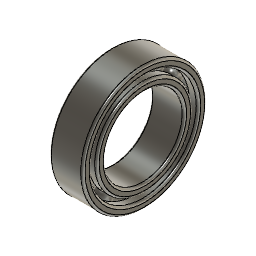
final (Autodesk Fusion 360 archive; units mm, degrees)
design "mr117zz"
Autodesk Fusion 360 part; units mm, degrees
sketch "Sketch1" plane through (0, 0, 0) normal (0, 0, 1) x (1, 0, 0)
  line L0 (-1.5, 3.5) -> (1.5, 3.5)
  line L1 (1.5, 3.5) -> (1.5, 4.25)
  line L2 (1.5, 4.25) -> (-1.5, 4.25)
  line L3 (-1.5, 4.25) -> (-1.5, 3.5)
  line L4 (-1.5, 5.5) -> (1.5, 5.5)
  line L5 (1.5, 5.5) -> (1.5, 4.75)
  line L6 (1.5, 4.75) -> (-1.5, 4.75)
  line L7 (-1.5, 4.75) -> (-1.5, 5.5)
  circle A0 centre (0, 4.5) radius 0.75
  line L8 (0, 3.5) -> (0, 5.5)
  line L9 (0, 3.5) -> (0, 0) construction
  dimension "d1" = 3
  dimension "d2" = 3.5
  dimension "d3" = 5.5
  dimension "d4" = 1.5
  dimension "d5" = 0.75
  constraint horizontal L0
  constraint vertical L1
  constraint horizontal L2
  constraint vertical L3
  constraint horizontal L4
  constraint vertical L5
  constraint horizontal L6
  constraint vertical L7
  constraint equal L0 L4
  constraint midpoint L0 L8.start
  constraint midpoint L4 L8.end
  constraint vertical L8
  constraint midpoint A0.centre L8
  constraint coincident L9.end origin
  constraint collinear L8 L9
  constraint equal L3 L7
  measures "d1" distance of L0.start L0.end
  measures "d2" distance of L9.end L0
  measures "d3" distance of L9.end L4
  measures "d4" diameter of A0
  measures "d5" distance of L0.start L2.end
revolve "Revolve1" add sketch "Sketch1" angle 360 about axis through (1.75, 0, 0) along (1, 0, 0) contours L0 L2 L3 A0 L8 | L0 L1 L2 A0 L8 | L4 L6 L7 A0 L8 | L4 L5 L6 A0 L8 makes body 1 at (-0.5, 3.4956, -0.1745) makes body 2 at (0.5, 5.4727, -0.5476)
revolve "Revolve2" add sketch "Sketch1" angle 360 about axis through (0, 3.5, 0) along (0, 1, 0) separate body contours L2 A0 L8 | L2 L6 A0 L8 | L6 A0 L8 picked at (-0.0341, 3.919) picked at (-0.2494, 4.483) picked at (-0.0341, 5.081) makes body 3
pattern_circular "C-Pattern1" count 12 over 360 about axis through (1.75, 0, 0) along (1, 0, 0) of bodies 3 makes body 4 at (-0.666, 4.2338, 2.3245) makes body 5 at (-0.666, 2.5043, 4.13) makes body 6 at (-0.666, 0.1038, 4.8288) makes body 7 at (-0.666, -2.3245, 4.2338) makes body 8 at (-0.666, -4.13, 2.5043) makes body 9 at (-0.666, -4.8288, 0.1038) makes body 10 at (-0.666, -4.2338, -2.3245) makes body 11 at (-0.666, -2.5043, -4.13) makes body 12 at (-0.666, -0.1038, -4.8288) makes body 13 at (-0.666, 2.5043, -4.13) makes body 14 at (-0.666, 4.13, -2.5043)
fillet "Fillet1" radius 0.2 4 faces at (1.5, 3.9842, -0.2111) (-1.5, 3.9842, -0.2111) (1.5, 5.2295, -0.2732) (-1.5, 5.2295, -0.2732) on bodies 1 2
copy_body "Body->Comp1" bodies 1 removing the originals makes body 15 in component "inner"
copy_body "Body->Comp2" bodies 2 removing the originals makes body 16 in component "outer"
copy_body "CutPasteBodies1" bodies 3 10 11 4 7 5 14 13 12 6 9 8 removing the originals makes body 17 makes body 18 makes body 19 makes body 20 makes body 21 makes body 22 makes body 23 makes body 24 makes body 25 makes body 26 makes body 27 makes body 28 in component "outer"
copy_body "CutPasteBodies1'" bodies 17 28 23 22 19 20 21 18 24 25 27 26 removing the originals makes body 29 makes body 30 makes body 31 makes body 32 makes body 33 makes body 34 makes body 35 makes body 36 makes body 37 makes body 38 makes body 39 makes body 40 in component "inner"
component "inner" placed x (1, 0, 0) y (0, 1, 0) z (0, 0, 1) at (0, 0, 0)
component "outer" placed x (1, 0, 0) y (0, 1, 0) z (0, 0, 1) at (0, 0, 0)
equation "d2 = ( 7 / 2 ) * 1 mm"
equation "d3 = ( 11 / 2 ) * 1 mm"

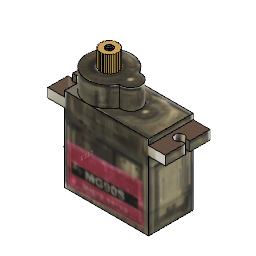
design "mg90s"
Autodesk Fusion 360 part; units mm, degrees
sketch "Shaft" plane through (0, 0, 0) normal (0, 1, 0) x (1, 0, 0) in component "Shaft"
  circle A0 centre (0, 0) radius 1
  circle A1 centre (0, 0) radius 2.4
  circle A2 centre (0, 0) radius 2.25 construction
  line L0 (0, 0) -> (0, 2.4) construction
  line L1 (0, 0) -> (-0.741641, 2.282536) construction
  line L2 (-0.695288, 2.139877) -> (0, 2.25) construction
  line L3 (-0.347644, 2.194939) -> (-0.375443, 2.370452) construction
  line L4 (0, 2.4) -> (-4, 2.4) construction
  line L5 (-0.351978, 2.222299) -> (-1.537204, 2.034577) construction
  spline S0 degree 5 poles (0, 2.4) (-0.019472, 2.4) (-0.055772, 2.396788) (-0.102302, 2.382342) (-0.151568, 2.347419) (-0.205208, 2.293022) (-0.253386, 2.253987) (-0.298375, 2.233713) (-0.333289, 2.225259) (-0.351978, 2.222299) knots 0 0 0 0 0 0 0.2 0.4 0.6 0.8 1 1 1 1 1 1
  line L6 (0.047124, 2.4) -> (-0.047124, 2.4)
  line L7 (-0.305434, 2.229671) -> (-0.398521, 2.214927)
  spline S1 degree 5 poles (0, 2.4) (0.019472, 2.4) (0.055772, 2.396788) (0.102302, 2.382342) (0.151568, 2.347419) (0.205208, 2.293022) (0.253386, 2.253987) (0.298375, 2.233713) (0.333289, 2.225259) (0.351978, 2.222299) knots 0 0 0 0 0 0 0.2 0.4 0.6 0.8 1 1 1 1 1 1
  line L8 (-0.047124, 2.4) -> (0.047124, 2.4)
  line L9 (0.305434, 2.229671) -> (0.398521, 2.214927)
  line L10 (0.351978, 2.222299) -> (0, 0)
  line L11 (-0.351978, 2.222299) -> (0, 0)
  circle A3 centre (0, 0) radius 1.625
  spline S2 degree 5 poles (-0.741641, 2.282536) (-0.723122, 2.288553) (-0.687606, 2.296715) (-0.638889, 2.297355) (-0.581243, 2.279365) (-0.513418, 2.244207) (-0.455536, 2.22197) (-0.406484, 2.21659) (-0.370666, 2.219339) (-0.351978, 2.222299) knots 0 0 0 0 0 0 0.2 0.4 0.6 0.8 1 1 1 1 1 1
  line L12 (-0.786458, 2.267974) -> (-0.696823, 2.297098)
  line L13 (-0.398521, 2.214927) -> (-0.305434, 2.229671)
  point P0 (-0.741641, 2.282536)
  point P1 (-1.410685, 1.941641)
  point P2 (-1.941641, 1.410685)
  point P3 (-2.282536, 0.741641)
  point P4 (-0.347644, 2.194939)
  point P5 (-2.4, 0)
  point P6 (-2.282536, -0.741641)
  point P7 (-1.941641, -1.410685)
  point P8 (-1.410685, -1.941641)
  point P9 (-0.741641, -2.282536)
  point P10 (0, -2.4)
  point P11 (0.741641, -2.282536)
  point P12 (1.410685, -1.941641)
  point P13 (1.941641, -1.410685)
  point P14 (2.282536, -0.741641)
  point P15 (2.4, 0)
  point P16 (2.282536, 0.741641)
  point P17 (1.941641, 1.410685)
  point P18 (1.410685, 1.941641)
  point P19 (0.741641, 2.282536)
  dimension "ScrewholeDia" = 2
  dimension "ShaftOuterDia" = 4.8
  dimension "ShaftSplinesInnerDia" = 4.5
  dimension "d5" = 360
  dimension "d6" = 4
  dimension "d7" = 1.2
  dimension "SplineTipPointiness" = 0.094248
  dimension "SplineInnerPointiness" = 0.094248
  dimension "d13" = 3.25
  constraint coincident A0.centre A1.centre
  constraint concentric A0 A1
  constraint concentric A0 A2
  constraint coincident A1 L0.end
  constraint vertical L0
  constraint coincident A2 L2.end
  constraint coincident L0 L2.end
  constraint perpendicular L2 L3
  constraint tangent A1 L4
  constraint perpendicular L3 L5
  constraint midpoint L0.end L6
  constraint parallel L4 L6
  constraint parallel L5 L7
  constraint symmetric L4.start L0 S0.start
  constraint concentric A1 A3
  measures "ScrewholeDia" diameter of A0
  measures "ShaftOuterDia" diameter of A1
  measures "ShaftSplinesInnerDia" diameter of A2
  measures "d6" distance of L0.end L4.end
  measures "d13" diameter of A3
extrude "Extrude3" add sketch "Shaft" against normal blind 4.5 contours A0 L10 L11 | A0 L10 L11 A3 | A0 L10 L11 | A0 L10 L11 A3 | S0 S1 L10 L11 A3 | A1 S1 L10 L11 A3 S2 | A1 S0 S2 picked at (0.524729, -0.4083) picked at (1.407237, -0.128115) picked at (0, 0.665753) picked at (-0.130529, 1.408799) picked at (-0.028349, 2.051428) picked at (-0.839001, 1.964928) picked at (-0.367278, 2.318902) makes body 1 in component "Shaft"
extrude "Extrude4" cut sketch "Shaft" against normal blind 4.5 contours A0 L10 L11 | A0 L10 L11 | A1 S0 S2 picked at (0.524729, -0.4083) picked at (0, 0.665753) picked at (-0.367278, 2.318902) bodies 1 in component "Shaft"
pattern_circular "C-Pattern3" count 20 over 360 about axis through (0, 1.75, 0) along (0, 1, 0) of "Extrude4" in component "Shaft"
extrude "Ignore" add sketch "Shaft" along normal blind 4.5 separate body contours A0 L10 L11 A3 | S0 S1 L10 L11 A3 picked at (-0.017445, 1.414725) picked at (0.028349, 2.051428) makes body 2 in component "Shaft"
coil "CoilPrimitive1" add diameter 2 section triangle in size 0.2 inside turns 11.25 pitch 0.4 right hand placed x (1, 0, 0) y (0, 0, 1) z (0, -1, 0) at (0, 0, 0) separate body makes body 3 in component "Shaft"
extrude "Extrude5" add sketch "Shaft" against normal blind 4.5 separate body contours A0 L10 L11 | A0 L10 L11 picked at (-0.54666, 0.378434) picked at (0.06959, 0.662106) makes body 4 in component "Shaft"
combine "Combine2" operation intersect target body 4 tool bodies 3 in component "Shaft"
sketch "Hat" plane through (0, -4.5, 0) normal (0, -1, 0) x (1, 0, 0) in component "Servo"
  circle A0 centre (0, 0) radius 1
  spline S0 degree 5 poles (0, -2.4) (0.019472, -2.4) (0.055772, -2.396788) (0.102302, -2.382342) (0.151568, -2.347419) (0.205208, -2.293022) (0.253386, -2.253987) (0.298375, -2.233713) (0.333289, -2.225259) (0.351978, -2.222299) knots 0 0 0 0 0 0 0.2 0.4 0.6 0.8 1 1 1 1 1 1
  spline S1 degree 5 poles (0.351978, -2.222299) (0.370666, -2.219339) (0.406484, -2.21659) (0.455536, -2.22197) (0.513418, -2.244207) (0.581243, -2.279365) (0.638889, -2.297355) (0.687606, -2.296715) (0.723122, -2.288553) (0.741641, -2.282536) knots -1 -1 -1 -1 -1 -1 -0.8 -0.6 -0.4 -0.2 0 0 0 0 0 0
  spline S2 degree 5 poles (0.741641, -2.282536) (0.760159, -2.276519) (0.79369, -2.262246) (0.833479, -2.234128) (0.869542, -2.185691) (0.903747, -2.117381) (0.937505, -2.065369) (0.974026, -2.032184) (1.004619, -2.013355) (1.021479, -2.004765) knots 0 0 0 0 0 0 0.2 0.4 0.6 0.8 1 1 1 1 1 1
  spline S3 degree 5 poles (1.021479, -2.004765) (1.038338, -1.996174) (1.071553, -1.982492) (1.119867, -1.972451) (1.181788, -1.975712) (1.257157, -1.988191) (1.317541, -1.987487) (1.363676, -1.971824) (1.394932, -1.953086) (1.410685, -1.941641) knots -1 -1 -1 -1 -1 -1 -0.8 -0.6 -0.4 -0.2 0 0 0 0 0 0
  spline S4 degree 5 poles (1.410685, -1.941641) (1.426437, -1.930196) (1.453917, -1.90626) (1.483069, -1.867223) (1.502399, -1.810012) (1.513821, -1.734476) (1.529854, -1.674577) (1.554334, -1.631731) (1.577611, -1.60437) (1.59099, -1.59099) knots 0 0 0 0 0 0 0.2 0.4 0.6 0.8 1 1 1 1 1 1
  spline S5 degree 5 poles (1.59099, -1.59099) (1.60437, -1.577611) (1.631731, -1.554334) (1.674577, -1.529854) (1.734476, -1.513821) (1.810012, -1.502399) (1.867223, -1.483069) (1.90626, -1.453917) (1.930196, -1.426437) (1.941641, -1.410685) knots -1 -1 -1 -1 -1 -1 -0.8 -0.6 -0.4 -0.2 0 0 0 0 0 0
  spline S6 degree 5 poles (1.941641, -1.410685) (1.953086, -1.394932) (1.971824, -1.363676) (1.987487, -1.317541) (1.988191, -1.257157) (1.975712, -1.181788) (1.972451, -1.119867) (1.982492, -1.071553) (1.996174, -1.038338) (2.004765, -1.021479) knots 0 0 0 0 0 0 0.2 0.4 0.6 0.8 1 1 1 1 1 1
  spline S7 degree 5 poles (2.004765, -1.021479) (2.013355, -1.004619) (2.032184, -0.974026) (2.065369, -0.937505) (2.117381, -0.903747) (2.185691, -0.869542) (2.234128, -0.833479) (2.262246, -0.79369) (2.276519, -0.760159) (2.282536, -0.741641) knots -1 -1 -1 -1 -1 -1 -0.8 -0.6 -0.4 -0.2 0 0 0 0 0 0
  spline S8 degree 5 poles (2.282536, -0.741641) (2.288553, -0.723122) (2.296715, -0.687606) (2.297355, -0.638889) (2.279365, -0.581243) (2.244207, -0.513418) (2.22197, -0.455536) (2.21659, -0.406484) (2.219339, -0.370666) (2.222299, -0.351978) knots 0 0 0 0 0 0 0.2 0.4 0.6 0.8 1 1 1 1 1 1
  spline S9 degree 5 poles (2.222299, -0.351978) (2.225259, -0.333289) (2.233713, -0.298375) (2.253987, -0.253386) (2.293022, -0.205208) (2.347419, -0.151568) (2.382342, -0.102302) (2.396788, -0.055772) (2.4, -0.019472) (2.4, 0) knots -1 -1 -1 -1 -1 -1 -0.8 -0.6 -0.4 -0.2 0 0 0 0 0 0
  spline S10 degree 5 poles (2.4, 0) (2.4, 0.019472) (2.396788, 0.055772) (2.382342, 0.102302) (2.347419, 0.151568) (2.293022, 0.205208) (2.253987, 0.253386) (2.233713, 0.298375) (2.225259, 0.333289) (2.222299, 0.351978) knots 0 0 0 0 0 0 0.2 0.4 0.6 0.8 1 1 1 1 1 1
  spline S11 degree 5 poles (2.222299, 0.351978) (2.219339, 0.370666) (2.21659, 0.406484) (2.22197, 0.455536) (2.244207, 0.513418) (2.279365, 0.581243) (2.297355, 0.638889) (2.296715, 0.687606) (2.288553, 0.723122) (2.282536, 0.741641) knots -1 -1 -1 -1 -1 -1 -0.8 -0.6 -0.4 -0.2 0 0 0 0 0 0
  spline S12 degree 5 poles (2.282536, 0.741641) (2.276519, 0.760159) (2.262246, 0.79369) (2.234128, 0.833479) (2.185691, 0.869542) (2.117381, 0.903747) (2.065369, 0.937505) (2.032184, 0.974026) (2.013355, 1.004619) (2.004765, 1.021479) knots 0 0 0 0 0 0 0.2 0.4 0.6 0.8 1 1 1 1 1 1
  spline S13 degree 5 poles (2.004765, 1.021479) (1.996174, 1.038338) (1.982492, 1.071553) (1.972451, 1.119867) (1.975712, 1.181788) (1.988191, 1.257157) (1.987487, 1.317541) (1.971824, 1.363676) (1.953086, 1.394932) (1.941641, 1.410685) knots -1 -1 -1 -1 -1 -1 -0.8 -0.6 -0.4 -0.2 0 0 0 0 0 0
  spline S14 degree 5 poles (1.941641, 1.410685) (1.930196, 1.426437) (1.90626, 1.453917) (1.867223, 1.483069) (1.810012, 1.502399) (1.734476, 1.513821) (1.674577, 1.529854) (1.631731, 1.554334) (1.60437, 1.577611) (1.59099, 1.59099) knots 0 0 0 0 0 0 0.2 0.4 0.6 0.8 1 1 1 1 1 1
  spline S15 degree 5 poles (1.59099, 1.59099) (1.577611, 1.60437) (1.554334, 1.631731) (1.529854, 1.674577) (1.513821, 1.734476) (1.502399, 1.810012) (1.483069, 1.867223) (1.453917, 1.90626) (1.426437, 1.930196) (1.410685, 1.941641) knots -1 -1 -1 -1 -1 -1 -0.8 -0.6 -0.4 -0.2 0 0 0 0 0 0
  spline S16 degree 5 poles (1.410685, 1.941641) (1.394932, 1.953086) (1.363676, 1.971824) (1.317541, 1.987487) (1.257157, 1.988191) (1.181788, 1.975712) (1.119867, 1.972451) (1.071553, 1.982492) (1.038338, 1.996174) (1.021479, 2.004765) knots 0 0 0 0 0 0 0.2 0.4 0.6 0.8 1 1 1 1 1 1
  spline S17 degree 5 poles (1.021479, 2.004765) (1.004619, 2.013355) (0.974026, 2.032184) (0.937505, 2.065369) (0.903747, 2.117381) (0.869542, 2.185691) (0.833479, 2.234128) (0.79369, 2.262246) (0.760159, 2.276519) (0.741641, 2.282536) knots -1 -1 -1 -1 -1 -1 -0.8 -0.6 -0.4 -0.2 0 0 0 0 0 0
  spline S18 degree 5 poles (0.741641, 2.282536) (0.723122, 2.288553) (0.687606, 2.296715) (0.638889, 2.297355) (0.581243, 2.279365) (0.513418, 2.244207) (0.455536, 2.22197) (0.406484, 2.21659) (0.370666, 2.219339) (0.351978, 2.222299) knots 0 0 0 0 0 0 0.2 0.4 0.6 0.8 1 1 1 1 1 1
  spline S19 degree 5 poles (0.351978, 2.222299) (0.333289, 2.225259) (0.298375, 2.233713) (0.253386, 2.253987) (0.205208, 2.293022) (0.151568, 2.347419) (0.102302, 2.382342) (0.055772, 2.396788) (0.019472, 2.4) (0, 2.4) knots -1 -1 -1 -1 -1 -1 -0.8 -0.6 -0.4 -0.2 0 0 0 0 0 0
  spline S20 degree 5 poles (0, 2.4) (-0.019472, 2.4) (-0.055772, 2.396788) (-0.102302, 2.382342) (-0.151568, 2.347419) (-0.205208, 2.293022) (-0.253386, 2.253987) (-0.298375, 2.233713) (-0.333289, 2.225259) (-0.351978, 2.222299) knots 0 0 0 0 0 0 0.2 0.4 0.6 0.8 1 1 1 1 1 1
  spline S21 degree 5 poles (-0.351978, 2.222299) (-0.370666, 2.219339) (-0.406484, 2.21659) (-0.455536, 2.22197) (-0.513418, 2.244207) (-0.581243, 2.279365) (-0.638889, 2.297355) (-0.687606, 2.296715) (-0.723122, 2.288553) (-0.741641, 2.282536) knots -1 -1 -1 -1 -1 -1 -0.8 -0.6 -0.4 -0.2 0 0 0 0 0 0
  spline S22 degree 5 poles (-0.741641, 2.282536) (-0.760159, 2.276519) (-0.79369, 2.262246) (-0.833479, 2.234128) (-0.869542, 2.185691) (-0.903747, 2.117381) (-0.937505, 2.065369) (-0.974026, 2.032184) (-1.004619, 2.013355) (-1.021479, 2.004765) knots 0 0 0 0 0 0 0.2 0.4 0.6 0.8 1 1 1 1 1 1
  spline S23 degree 5 poles (-1.021479, 2.004765) (-1.038338, 1.996174) (-1.071553, 1.982492) (-1.119867, 1.972451) (-1.181788, 1.975712) (-1.257157, 1.988191) (-1.317541, 1.987487) (-1.363676, 1.971824) (-1.394932, 1.953086) (-1.410685, 1.941641) knots -1 -1 -1 -1 -1 -1 -0.8 -0.6 -0.4 -0.2 0 0 0 0 0 0
  spline S24 degree 5 poles (-1.410685, 1.941641) (-1.426437, 1.930196) (-1.453917, 1.90626) (-1.483069, 1.867223) (-1.502399, 1.810012) (-1.513821, 1.734476) (-1.529854, 1.674577) (-1.554334, 1.631731) (-1.577611, 1.60437) (-1.59099, 1.59099) knots 0 0 0 0 0 0 0.2 0.4 0.6 0.8 1 1 1 1 1 1
  spline S25 degree 5 poles (-1.59099, 1.59099) (-1.60437, 1.577611) (-1.631731, 1.554334) (-1.674577, 1.529854) (-1.734476, 1.513821) (-1.810012, 1.502399) (-1.867223, 1.483069) (-1.90626, 1.453917) (-1.930196, 1.426437) (-1.941641, 1.410685) knots -1 -1 -1 -1 -1 -1 -0.8 -0.6 -0.4 -0.2 0 0 0 0 0 0
  spline S26 degree 5 poles (-1.941641, 1.410685) (-1.953086, 1.394932) (-1.971824, 1.363676) (-1.987487, 1.317541) (-1.988191, 1.257157) (-1.975712, 1.181788) (-1.972451, 1.119867) (-1.982492, 1.071553) (-1.996174, 1.038338) (-2.004765, 1.021479) knots 0 0 0 0 0 0 0.2 0.4 0.6 0.8 1 1 1 1 1 1
  spline S27 degree 5 poles (-2.004765, 1.021479) (-2.013355, 1.004619) (-2.032184, 0.974026) (-2.065369, 0.937505) (-2.117381, 0.903747) (-2.185691, 0.869542) (-2.234128, 0.833479) (-2.262246, 0.79369) (-2.276519, 0.760159) (-2.282536, 0.741641) knots -1 -1 -1 -1 -1 -1 -0.8 -0.6 -0.4 -0.2 0 0 0 0 0 0
  spline S28 degree 5 poles (-2.282536, 0.741641) (-2.288553, 0.723122) (-2.296715, 0.687606) (-2.297355, 0.638889) (-2.279365, 0.581243) (-2.244207, 0.513418) (-2.22197, 0.455536) (-2.21659, 0.406484) (-2.219339, 0.370666) (-2.222299, 0.351978) knots 0 0 0 0 0 0 0.2 0.4 0.6 0.8 1 1 1 1 1 1
  spline S29 degree 5 poles (-2.222299, 0.351978) (-2.225259, 0.333289) (-2.233713, 0.298375) (-2.253987, 0.253386) (-2.293022, 0.205208) (-2.347419, 0.151568) (-2.382342, 0.102302) (-2.396788, 0.055772) (-2.4, 0.019472) (-2.4, 0) knots -1 -1 -1 -1 -1 -1 -0.8 -0.6 -0.4 -0.2 0 0 0 0 0 0
  spline S30 degree 5 poles (-2.4, 0) (-2.4, -0.019472) (-2.396788, -0.055772) (-2.382342, -0.102302) (-2.347419, -0.151568) (-2.293022, -0.205208) (-2.253987, -0.253386) (-2.233713, -0.298375) (-2.225259, -0.333289) (-2.222299, -0.351978) knots 0 0 0 0 0 0 0.2 0.4 0.6 0.8 1 1 1 1 1 1
  spline S31 degree 5 poles (-2.222299, -0.351978) (-2.219339, -0.370666) (-2.21659, -0.406484) (-2.22197, -0.455536) (-2.244207, -0.513418) (-2.279365, -0.581243) (-2.297355, -0.638889) (-2.296715, -0.687606) (-2.288553, -0.723122) (-2.282536, -0.741641) knots -1 -1 -1 -1 -1 -1 -0.8 -0.6 -0.4 -0.2 0 0 0 0 0 0
  spline S32 degree 5 poles (-2.282536, -0.741641) (-2.276519, -0.760159) (-2.262246, -0.79369) (-2.234128, -0.833479) (-2.185691, -0.869542) (-2.117381, -0.903747) (-2.065369, -0.937505) (-2.032184, -0.974026) (-2.013355, -1.004619) (-2.004765, -1.021479) knots 0 0 0 0 0 0 0.2 0.4 0.6 0.8 1 1 1 1 1 1
  spline S33 degree 5 poles (-2.004765, -1.021479) (-1.996174, -1.038338) (-1.982492, -1.071553) (-1.972451, -1.119867) (-1.975712, -1.181788) (-1.988191, -1.257157) (-1.987487, -1.317541) (-1.971824, -1.363676) (-1.953086, -1.394932) (-1.941641, -1.410685) knots -1 -1 -1 -1 -1 -1 -0.8 -0.6 -0.4 -0.2 0 0 0 0 0 0
  spline S34 degree 5 poles (-1.941641, -1.410685) (-1.930196, -1.426437) (-1.90626, -1.453917) (-1.867223, -1.483069) (-1.810012, -1.502399) (-1.734476, -1.513821) (-1.674577, -1.529854) (-1.631731, -1.554334) (-1.60437, -1.577611) (-1.59099, -1.59099) knots 0 0 0 0 0 0 0.2 0.4 0.6 0.8 1 1 1 1 1 1
  spline S35 degree 5 poles (-1.59099, -1.59099) (-1.577611, -1.60437) (-1.554334, -1.631731) (-1.529854, -1.674577) (-1.513821, -1.734476) (-1.502399, -1.810012) (-1.483069, -1.867223) (-1.453917, -1.90626) (-1.426437, -1.930196) (-1.410685, -1.941641) knots -1 -1 -1 -1 -1 -1 -0.8 -0.6 -0.4 -0.2 0 0 0 0 0 0
  spline S36 degree 5 poles (-1.410685, -1.941641) (-1.394932, -1.953086) (-1.363676, -1.971824) (-1.317541, -1.987487) (-1.257157, -1.988191) (-1.181788, -1.975712) (-1.119867, -1.972451) (-1.071553, -1.982492) (-1.038338, -1.996174) (-1.021479, -2.004765) knots 0 0 0 0 0 0 0.2 0.4 0.6 0.8 1 1 1 1 1 1
  spline S37 degree 5 poles (-1.021479, -2.004765) (-1.004619, -2.013355) (-0.974026, -2.032184) (-0.937505, -2.065369) (-0.903747, -2.117381) (-0.869542, -2.185691) (-0.833479, -2.234128) (-0.79369, -2.262246) (-0.760159, -2.276519) (-0.741641, -2.282536) knots -1 -1 -1 -1 -1 -1 -0.8 -0.6 -0.4 -0.2 0 0 0 0 0 0
  spline S38 degree 5 poles (-0.741641, -2.282536) (-0.723122, -2.288553) (-0.687606, -2.296715) (-0.638889, -2.297355) (-0.581243, -2.279365) (-0.513418, -2.244207) (-0.455536, -2.22197) (-0.406484, -2.21659) (-0.370666, -2.219339) (-0.351978, -2.222299) knots 0 0 0 0 0 0 0.2 0.4 0.6 0.8 1 1 1 1 1 1
  spline S39 degree 5 poles (-0.351978, -2.222299) (-0.333289, -2.225259) (-0.298375, -2.233713) (-0.253386, -2.253987) (-0.205208, -2.293022) (-0.151568, -2.347419) (-0.102302, -2.382342) (-0.055772, -2.396788) (-0.019472, -2.4) (0, -2.4) knots -1 -1 -1 -1 -1 -1 -0.8 -0.6 -0.4 -0.2 0 0 0 0 0 0
  circle A1 centre (0, 0) radius 6
  line L0 (0, 0) -> (-6, 0) construction
  line L1 (-6, 0) -> (8.5, 0) construction
  circle A2 centre (5.75, 0) radius 2.75
  line L2 (8.5, 0) -> (5.75, 0) construction
  dimension "HatDia" = 12
  dimension "HatTipDia" = 5.5
  dimension "d36" = 2.75
  dimension "HornCollarDepth" = -2.7
  dimension "HornUnderside" = -1
  dimension "HornInnerScrewTabThickness" = 1.2
  dimension "HornUpperHeight" = 2.3
  dimension "ServoTrayThickness" = 3
  constraint concentric A0 A1
  constraint coincident A0.centre A1.centre
  constraint coincident A1 L0.end
  constraint horizontal L0
  constraint parallel L0 L1
  constraint parallel L1 L2
  constraint coincident A2.centre L2.end
  measures "HatDia" diameter of A1
  measures "HatTipDia" diameter of A2
  measures "d36" distance of L1.end A2.centre
extrude "Extrude1" add sketch "Hat" along normal blind 5.5 separate body contours S0 S1 S2 S3 S4 S5 S6 S7 S8 S9 S10 S11 S12 S13 S14 S15 S16 S17 S18 S19 S20 S21 S22 S23 S24 S25 S26 S27 S28 S29 S30 S31 S32 S33 S34 S35 S36 S37 S38 S39 | A1 A2 | A1 A2 | A1 A2 picked at (1.828362, 0.000863) picked at (5.009249, -0.439125) picked at (6.782206, -0.493586) picked at (2.982895, -2.906238) makes body 5 in component "Servo"
sketch "ServoBody" plane through (0, -10, 0) normal (0, -1, 0) x (1, 0, 0) in component "Servo"
  line L0 (0, 0) -> (-6, 0) construction
  line L1 (-6, 0) -> (16.5, 0) construction
  line L2 (16.5, 0) -> (16.5, 12)
  line L3 (16.5, 6) -> (-6, 6)
  line L4 (-6, 6) -> (-6, 0)
  line L5 (16.5, 0) -> (16.5, -12)
  line L6 (16.5, -6) -> (-6, -6)
  line L7 (-6, -6) -> (-6, 0)
  circle A0 centre (0, 0) radius 1
  arc A1 (5.347826, -2.720433) -> (5.347826, 2.720433) centre (5.75, 0) ccw
  arc A2 (5.347826, 2.720433) -> (5.347826, -2.720433) centre (0, 0) ccw
  dimension "Hole_to_closest_end_dist" = 6
  dimension "ServoBodyLength" = 22.5
  dimension "ServoBodyWidth" = 12
  constraint coincident L0.start A0.centre
  constraint horizontal L0
  constraint parallel L0 L1
  constraint perpendicular L1 L2
  constraint midpoint L2 L3.start
  constraint perpendicular L2 L3
  constraint perpendicular L1 L4
  constraint symmetric L0.end L1 L4.end
  constraint symmetric L2.start L1 L5.start
  constraint symmetric L1 L2.end L5.end
  constraint symmetric L1 L3.start L6.start
  constraint symmetric L1 L3.end L6.end
  measures "Hole_to_closest_end_dist" distance of L0.start L0.end
  measures "ServoBodyLength" distance of L0.end L1.end
  measures "ServoBodyWidth" distance of L1.end L2.end
extrude "Extrude2" add sketch "ServoBody" along normal blind 22.5 contours L2 L3 L5 L6 A1 A2 | L3 L4 A2 | A1 A2 | L6 L7 A2 | A0 picked at (13.770173, 2.334371) picked at (-4.821221, 4.821221) picked at (3.898551, 0) picked at (-4.821221, -4.821221) picked at (-0.32961, 0.503129) bodies 5 in component "Servo"
ref_plane "WorkPlane1" through (8.25, -11.5, 0) normal (0, 1, 0) x (-1, 0, 0) in component "Servo"
sketch "ScrewTab" plane through (5.45, -11.5, 0) normal (0, 1, 0) x (1, 0, 0) in component "Servo"
  line L0 (11.05, -6) -> (-11.45, -6)
  line L1 (-11.45, -6) -> (-11.45, 0)
  line L2 (-11.45, 6) -> (-11.45, 0)
  line L3 (11.05, 6) -> (-11.45, 6)
  line L4 (11.05, 0) -> (11.05, 12)
  line L5 (11.05, 0) -> (11.05, -12)
  line L6 (-11.45, 0) -> (11.05, 0)
  line L7 (-11.45, -6) -> (-15.95, -6)
  line L8 (-15.95, -6) -> (-15.95, 6) construction
  line L9 (-15.95, 6) -> (-11.45, 6)
  line L10 (-11.45, 6) -> (-11.45, -6)
  line L11 (11.05, -6) -> (15.55, -6)
  line L12 (15.55, -6) -> (15.55, 6) construction
  line L13 (15.55, 6) -> (11.05, 6)
  line L14 (11.05, 6) -> (11.05, -6)
  line L15 (15.55, 0) -> (12, 0) construction
  circle A0 centre (13.3, 0) radius 1.3
  line L16 (12, 0) -> (13.3, 0) construction
  line L17 (15.55, 0) -> (-15.95, 0) construction
  line L18 (-0.2, 0) -> (-0.2, -6) construction
  line L19 (15.55, -6) -> (15.55, -0.6)
  line L20 (15.55, -0.6) -> (14.453256, -0.6)
  line L21 (15.55, 0.6) -> (14.453256, 0.6)
  line L22 (15.55, 6) -> (15.55, 0.6)
  circle A1 centre (-13.7, 0) radius 1.3
  line L23 (-15.95, 0.6) -> (-14.853256, 0.6)
  line L24 (-15.95, -0.6) -> (-14.853256, -0.6)
  line L25 (-15.95, -6) -> (-15.95, -0.6)
  line L26 (-15.95, 6) -> (-15.95, 0.6)
  line L27 (11.05, 0) -> (15.55, 0) construction
  dimension "ServoTabSize" = 4.5
  dimension "d47" = 12
  dimension "d48" = 4.5
  dimension "d49" = 12
  dimension "TabScrewSize" = 2.6
  dimension "d52" = 1.3
  dimension "d53" = 6
  dimension "d55" = 5.4
  dimension "HornArmTopSide" = -1.5
  constraint horizontal L7
  constraint vertical L8
  constraint horizontal L9
  constraint vertical L10
  constraint coincident L0.end L1.start
  constraint horizontal L11
  constraint vertical L12
  constraint horizontal L13
  constraint vertical L14
  constraint coincident L0.start L11.start
  constraint midpoint L12 L15.start
  constraint perpendicular L12 L15
  constraint perpendicular L12 L16
  constraint coincident A0.centre L16.end
  constraint midpoint L8 L17.end
  constraint coincident L6 L18.start
  constraint perpendicular L6 L18
  constraint midpoint L17 L18.start
  constraint perpendicular L11 L19
  constraint perpendicular L19 L20
  constraint symmetric L11.end L15 L12.end
  constraint symmetric L15 L19.end L21.start
  constraint symmetric L11.end L18 L7.end
  constraint symmetric A0 L18 A1
  constraint symmetric L18 L19.end L24.start
  constraint symmetric L18 L21.start L23.start
  constraint symmetric L18 L12.end L8.end
  constraint coincident L4.start L5.start
  constraint midpoint A0.centre L27
  measures "ServoTabSize" distance of L0.end L7.end
  measures "d47" distance of L0.end L2.start
  measures "d48" distance of L0.start L11.end
  measures "d49" distance of L0.start L3.start
  measures "TabScrewSize" diameter of A0
  measures "d52" distance of L15.end A0.centre
  measures "d53" distance of L18.start L18.end
  measures "d55" distance of L11.end L19.end
extrude "Extrude3'" add sketch "ScrewTab" against normal blind 2.5 contours L4 L5 L11 L13 L14 A0 L19 L20 L21 L22 | L1 L2 L7 L9 L10 A1 L23 L24 L25 L26 picked at (13.32421, -4.432657) picked at (-13.72421, 4.432657) bodies 5 in component "Servo"
sketch "WireHole" plane through (-6, 0, 0) normal (-1, 0, 0) x (0, 0, 1) in component "Servo"
  line L0 (-6, -17.324116) -> (-6, -18.73833) construction
  line L1 (-6, -18.73833) -> (6, -18.73833) construction
  line L2 (6, -17.324116) -> (-6, -17.324116)
  line L3 (6, -17.324116) -> (-6, -17.324116) construction
  line L4 (-6, -18.73833) -> (6, -18.73833) construction
  line L5 (0, -28.5) -> (0, -27.5) construction
  line L6 (0, -27.5) -> (-1.5, -27.5)
  line L7 (-1.5, -27.5) -> (1.5, -27.5)
  line L8 (1.5, -27.5) -> (1.5, -28.5)
  line L9 (1.5, -28.5) -> (-1.5, -28.5)
  line L10 (-1.5, -28.5) -> (-1.5, -27.5)
  line L11 (1.5, -28) -> (-1.5, -28) construction
  circle A0 centre (0, -28) radius 0.375
  line L12 (0, -28) -> (-0.85, -28) construction
  circle A1 centre (-0.85, -28) radius 0.375
  circle A2 centre (0.85, -28) radius 0.375
  line L13 (6, -14) -> (-6, -14)
  line L14 (-6, -14) -> (-6, -32.5)
  line L15 (-6, -32.5) -> (6, -32.5)
  line L16 (6, -32.5) -> (6, -14)
  line L17 (0, -32.5) -> (0, -14) construction
  dimension "d61" = 1
  dimension "d62" = 1.5
  dimension "d63" = 3
  dimension "d64" = 1
  dimension "d65" = 0.75
  dimension "d66" = 0.85
  dimension "d67" = 0.75
  dimension "d133" = 4
  constraint perpendicular L1 L5
  constraint perpendicular L5 L6
  constraint horizontal L7
  constraint vertical L8
  constraint horizontal L9
  constraint vertical L10
  constraint midpoint L8 L11.start
  constraint midpoint L10 L11.end
  constraint midpoint L5 A0.centre
  constraint coincident A0.centre L12.start
  constraint perpendicular L5 L12
  constraint coincident L12.end A1.centre
  constraint symmetric L5 A1 A2
  constraint midpoint L15 L17.start
  constraint midpoint L13 L17.end
  constraint coincident A0.centre L17
  measures "d61" distance of L5.start L5.end
  measures "d62" distance of L5.end L6.end
  measures "d63" distance of L6.end L7.end
  measures "d64" distance of L6.end L9.end
  measures "d65" diameter of A0
  measures "d66" distance of A0.centre L12.end
  measures "d67" diameter of A1
  measures "d133" distance of L9 L15
extrude "Extrude4'" cut sketch "WireHole" against normal blind 3 contours L6 L7 L8 L9 L10 picked at (1.408333, -28) bodies 5 in component "Servo"
extrude "Extrude5'" add sketch "WireHole" along normal blind 5 separate body contours A0 | A1 | A2 picked at (0.091631, -27.84129) picked at (-0.74672, -27.892324) picked at (0.95328, -27.892324) makes body 6 at (-9.333333, -28.092534, -1.213404) makes body 7 at (-9.333333, -27.871742, 0.352385) makes body 8 at (-9.333333, -28.092534, 0.486596) in component "Servo"
sketch "ServoOrigin" plane through (0, 0, 0) normal (0, 1, 0) x (-1, 0, 0) in component "Servo"
  circle A0 centre (0, 0) radius 1
sketch "Sketch1" plane through (0, 0, 0) normal (0, 1, 0) x (-1, 0, 0) in component "Joint"
  circle A0 centre (0, 0) radius 1
sketch "Sketch1 (2)" plane through (0, -10, 0) normal (0, 1, 0) x (-1, 0, 0)
  circle A0 centre (0, 0) radius 1
  constraint coincident A0.centre origin
component "Servo" placed x (1, 0, 0) y (0, 1, 0) z (0, 0, 1) at (0, 0, 0)
component "Shaft" placed x (1, 0, 0) y (0, 1, 0) z (0, 0, 1) at (0, 0, 0) in component "Servo"
component "Joint" placed x (1, 0, 0) y (0, 1, 0) z (0, 0, 1) at (0, 0, 0) in component "Servo"
hidden bodies 2
equation "NumSplines = 20"
equation "d7 = ShaftOuterDia / 4"
equation "SplineTipPointiness = ShaftOuterDia * PI / NumSplines / 8"
equation "SplineInnerPointiness = ShaftOuterDia * PI / NumSplines / 8"
equation "ShaftHeight = 4.5 mm"
equation "d13 = ScrewholeDia + 0.5 * ( ( ShaftSplinesInnerDia - ScrewholeDia ) )"
equation "d20 = -ShaftHeight"
equation "d22 = -ShaftHeight"
equation "d24 = NumSplines"
equation "d26 = ScrewholeDia"
equation "ShaftScrewSectionsize = 0.2 mm"
equation "ShaftScrewPitch = ShaftHeight / 0.4 mm"
equation "d30 = -ShaftHeight"
equation "d31 = -ShaftHeight"
equation "n = 14.5 mm"
equation "d36 = HatTipDia / 2"
equation "HatHeight = 5.5 mm"
equation "Hole_to_closest_end_dist = HatDia / 2"
equation "ServoBodyHeight = 22.5 mm"
equation "ServoCornerWireRecess = 1 mm"
equation "ServoTabRecess = -1.5 mm"
equation "d47 = ServoBodyWidth"
equation "d49 = ServoBodyWidth"
equation "ServoHoleRecess = 3.6 mm"
equation "d52 = TabScrewSize / 2"
equation "d53 = ServoBodyWidth / 2"
equation "TabScrewGapSize = 1.2 mm"
equation "d55 = ( ServoBodyWidth - TabScrewGapSize ) / 2"
equation "TabThickness = -2.5 mm"
equation "WireHoleWidth = 3 mm"
equation "WireHoleOffset = 0.4 mm"
equation "WireHoleHeight = 1 mm"
equation "d61 = WireHoleHeight"
equation "d62 = WireHoleWidth / 2"
equation "d63 = WireHoleWidth"
equation "d64 = WireHoleHeight"
equation "d65 = WireHoleWidth / 4"
equation "d66 = WireHoleWidth / 4 + 0.1 mm"
equation "d67 = WireHoleWidth / 4"
equation "d68 = -WireHoleWidth"
equation "WireLenght = 5 mm"
equation "OuterHubDia = 7.3 mm + 2 * tol"
equation "InnerHubDia = 4.65 mm"
equation "MajorArmLen = 36.2 mm + 2 * tol"
equation "MinroArmLen = 19 mm + 2 * tol"
equation "TipDiaMajor = 5 mm + 2 * tol"
equation "TipDiaMinor = 4 mm + 2 * tol"
equation "ScrewHole = 2.5 mm"
equation "DriveHole = 2 mm"
equation "d14 = DriveHole"
equation "d19 = OuterHubDia + 1.5 mm + tol + 2 * tol"
equation "ReinforcerWidth = 1 mm + 2 * tol"
equation "HoleSlideAdj = 0.6 mm"
equation "SideHoleSlideAdj = 0.25 mm"
equation "TrayGap = 0.2 mm"
equation "TraySideWidth = 3 mm"
equation "TrayEndExtraMinus1 = 1 mm - TrayGap"
equation "d90 = OuterHubDia + 2 * tol"
equation "d92 = ReinforcerWidth / 2 + tol"
equation "d103 = HornUpperHeight / 3"
equation "d123 = TrayGap"
equation "d124 = TrayGap"
equation "d125 = TrayGap"
equation "d127 = TrayGap"
named bodies: "Ignore", "Shaft", "Thread", "Signal", "Positive", "Ground"
